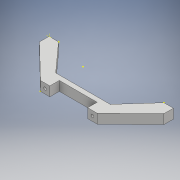
# Autodesk Inventor part: PosteV
Saved by Autodesk Inventor 2017 SP1 (Build 210196100, 196)
## iProperties
Part Number: PosteV
Material: Genérico
Document SubType Name: Modeling
Designer: Juan
Density: 1 g/cm^3
Appearance: Valor por defecto
Author: Juan
Autodesk Inventor part; units mm, degrees
sketch "Boceto1" plane through (0, 0, 0) normal (0, 0, 1) x (1, 0, 0)
  line L0 (-35.782, 44.9234) -> (-25.782, 44.9234)
  line L1 (-35.782, 44.9234) -> (-35.782, 34.9234)
  line L2 (-35.782, 34.9234) -> (0, 0)
  line L3 (0, 0) -> (10, 0)
  line L4 (10, 0) -> (10, 10)
  line L5 (10, 10) -> (30, 10)
  line L6 (30, 10) -> (30, 15)
  line L7 (30, 15) -> (1.1611, 15)
  line L8 (1.1611, 15) -> (-25.782, 44.9234)
  line L9 (95.782, 44.9234) -> (85.782, 44.9234)
  line L10 (95.782, 44.9234) -> (95.782, 34.9234)
  line L11 (95.782, 34.9234) -> (60, 0)
  line L12 (60, 0) -> (50, 0)
  line L13 (50, 0) -> (50, 10)
  line L14 (50, 10) -> (30, 10)
  line L15 (30, 15) -> (58.8389, 15)
  line L16 (58.8389, 15) -> (85.782, 44.9234)
  dimension "d0" = 10
  dimension "d1" = 10
  dimension "d2" = 50
  dimension "d3" = 10
  dimension "d4" = 10
  dimension "d5" = 20
  dimension "d6" = 5
  dimension "d9" = 132
  dimension "d10" = 40.2659
  dimension "d11" = 28.8389
  dimension "d54" = 132
  constraints: 34 end point, 7 symmetric about line, 5 perpendicular, 1 coincident, 1 horizontal, 1 vertical
  measures "d0" distance of L0.start L0.end
  measures "d1" distance of L0.start L1.end
  measures "d2" distance of L1.end L2.end
  measures "d3" distance of L2.end L3.end
  measures "d4" distance of L3.end L4.end
  measures "d5" distance of L4.end L5.end
  measures "d6" distance of L5.end L6.end
  measures "d9" angle of L7 L8
  measures "d10" distance of L7.end L0.end
  measures "d11" distance of L6.end L7.end
  measures "d54" angle of L15 L16
extrude "Extrusión1" add sketch "Boceto1" along normal blind 10
ref_plane "Plano de trabajo1" through (-35.782, 44.9234, 0) normal (0, 1, 0) x (1, 0, 0)
sketch "Boceto2" plane through (-35.782, 44.9234, 0) normal (0, 1, 0) x (1, 0, 0)
  point P0 (35.782, 0)
  point P1 (0, -10)
  point P2 (10, -10)
hole "Agujero1" at (-30.7761, 44.9234, 5.0015) direction (0, -1, 0) diameter 3 depth 5 tip angle 118
ref_plane "Plano de trabajo2" through (85.782, 44.9234, 0) normal (0, 1, 0) x (1, 0, 0)
sketch "Boceto3" plane through (85.782, 44.9234, 0) normal (0, 1, 0) x (1, 0, 0)
  point P0 (-85.782, 0)
  point P1 (0, -10)
hole "Agujero2" at (90.7683, 44.9234, 4.9912) direction (0, -1, 0) diameter 3 depth 5 tip angle 118
ref_plane "Plano de trabajo3" through (0, 0, 0) normal (0, -1, 0) x (1, 0, 0)
sketch "Boceto4" plane through (0, 0, 0) normal (0, -1, 0) x (1, 0, 0)
  point P0 (0, 0)
hole "Agujero3" at (4.993, 0, 5.0183) direction (0, 1, 0) diameter 3 depth 5 tip angle 118
ref_plane "Plano de trabajo4" through (50, 0, 0) normal (0, -1, 0) x (1, 0, 0)
sketch "Boceto5" plane through (50, 0, 0) normal (0, -1, 0) x (1, 0, 0)
  point P0 (-50, 0)
sketch "Boceto6" plane through (50, 0, 0) normal (0, -1, 0) x (1, 0, 0)
  point P0 (-50, 0)
hole "Agujero4" at (54.9983, 0, 5.0092) direction (0, 1, 0) diameter 3 depth 5 tip angle 118
sketch "Boceto7" plane through (85.782, 44.9234, 0) normal (0, 1, 0) x (1, 0, 0)
  point P0 (-85.782, 0)
sketch "Boceto8" plane through (50, 0, 0) normal (0, -1, 0) x (1, 0, 0)
  point P0 (-50, 0)
